Autodesk Fusion 360 part; units mm, degrees
note: some values were not read from the file. Set by a fixed rule: which sketch regions a step uses.
(part 17 of 20)
  spline S97 degree 5 poles (-21.1029, 22.7084) (-21.1018, 22.7059) (-21.0998, 22.7009) (-21.0967, 22.6934) (-21.0925, 22.6834) (-21.0873, 22.671) (-21.0822, 22.6586) (-21.077, 22.6462) (-21.0718, 22.6339) (-21.0666, 22.6217) (-21.0614, 22.6094) (-21.0562, 22.5972) (-21.051, 22.585) (-21.0458, 22.5729) (-21.0406, 22.5608) (-21.0354, 22.5487) (-21.0302, 22.5367) (-21.025, 22.5247) (-21.0198, 22.5127) (-21.0145, 22.5008) (-21.0093, 22.4889) (-21.0041, 22.4771) (-20.9989, 22.4653) (-20.9937, 22.4535) (-20.9884, 22.4417) (-20.9832, 22.43) (-20.978, 22.4184) (-20.9727, 22.4067) (-20.9675, 22.3951) (-20.9623, 22.3836) (-20.957, 22.3721) (-20.9518, 22.3606) (-20.9466, 22.3491) (-20.9413, 22.3377) (-20.9361, 22.3264) (-20.9308, 22.315) (-20.9256, 22.3037) (-20.9204, 22.2925) (-20.9151, 22.2812) (-20.9099, 22.2701) (-20.9046, 22.2589) (-20.8994, 22.2478) (-20.8942, 22.2367) (-20.8889, 22.2257) (-20.8837, 22.2147) (-20.8784, 22.2038) (-20.8732, 22.1928) (-20.868, 22.182) (-20.8627, 22.1711) (-20.8575, 22.1603) (-20.8523, 22.1496) (-20.847, 22.1388) (-20.8418, 22.1281) (-20.8366, 22.1175) (-20.8313, 22.1069) (-20.8261, 22.0963) (-20.8209, 22.0858) (-20.8157, 22.0753) (-20.8105, 22.0649) (-20.8052, 22.0544) (-20.8, 22.0441) (-20.7948, 22.0337) (-20.7896, 22.0235) (-20.7844, 22.0132) (-20.7792, 22.003) (-20.774, 21.9928) (-20.7688, 21.9827) (-20.7636, 21.9726) (-20.7584, 21.9625) (-20.7532, 21.9525) (-20.748, 21.9426) (-20.7429, 21.9326) (-20.7377, 21.9228) (-20.7325, 21.9129) (-20.7274, 21.9031) (-20.7222, 21.8933) (-20.717, 21.8836) (-20.7119, 21.8739) (-20.7067, 21.8643) (-20.7016, 21.8547) (-20.6965, 21.8451) (-20.6913, 21.8356) (-20.6862, 21.8261) (-20.6811, 21.8167) (-20.676, 21.8073) (-20.6709, 21.798) (-20.6658, 21.7887) (-20.6607, 21.7794) (-20.6556, 21.7702) (-20.6505, 21.761) (-20.6454, 21.7519) (-20.6404, 21.7428) (-20.6353, 21.7337) (-20.6303, 21.7247) (-20.6252, 21.7158) (-20.6202, 21.7068) (-20.6152, 21.698) (-20.6101, 21.6891) (-20.6051, 21.6803) (-20.6001, 21.6716) (-20.5951, 21.6629) (-20.5902, 21.6542) (-20.5852, 21.6456) (-20.5802, 21.6371) (-20.5753, 21.6285) (-20.5703, 21.6201) (-20.5654, 21.6116) (-20.5605, 21.6032) (-20.5555, 21.5949) (-20.5506, 21.5866) (-20.5457, 21.5783) (-20.5409, 21.5701) (-20.536, 21.5619) (-20.5311, 21.5538) (-20.5263, 21.5458) (-20.5214, 21.5377) (-20.5166, 21.5297) (-20.5118, 21.5218) (-20.507, 21.5139) (-20.5022, 21.5061) (-20.4974, 21.4983) (-20.4927, 21.4905) (-20.4879, 21.4828) (-20.4832, 21.4752) (-20.4784, 21.4676) (-20.4737, 21.46) (-20.469, 21.4525) (-20.4644, 21.445) (-20.4597, 21.4376) (-20.455, 21.4302) (-20.4504, 21.4229) (-20.4458, 21.4156) (-20.4412, 21.4084) (-20.4366, 21.4012) (-20.432, 21.3941) (-20.4274, 21.387) (-20.4229, 21.38) (-20.4184, 21.373) (-20.4139, 21.3661) (-20.4094, 21.3592) (-20.4049, 21.3523) (-20.4004, 21.3455) (-20.396, 21.3388) (-20.3916, 21.3321) (-20.3872, 21.3255) (-20.3828, 21.3189) (-20.3784, 21.3124) (-20.3741, 21.3059) (-20.3698, 21.2995) (-20.3655, 21.2931) (-20.3612, 21.2867) (-20.3569, 21.2805) (-20.3527, 21.2742) (-20.3484, 21.2681) (-20.3442, 21.2619) (-20.3401, 21.2559) (-20.3359, 21.2498) (-20.3318, 21.2439) (-20.3277, 21.238) (-20.3236, 21.2321) (-20.3195, 21.2263) (-20.3155, 21.2205) (-20.3115, 21.2148) (-20.3075, 21.2092) (-20.3035, 21.2036) (-20.2996, 21.1981) (-20.2956, 21.1926) (-20.2918, 21.1871) (-20.2879, 21.1818) (-20.2841, 21.1764) (-20.2802, 21.1712) (-20.2765, 21.166) (-20.2727, 21.1608) (-20.269, 21.1557) (-20.2653, 21.1507) (-20.2616, 21.1457) (-20.258, 21.1408) (-20.2544, 21.1359) (-20.2508, 21.1311) (-20.2472, 21.1263) (-20.2437, 21.1216) (-20.2402, 21.117) (-20.2368, 21.1124) (-20.2333, 21.1079) (-20.23, 21.1034) (-20.2266, 21.099) (-20.2233, 21.0947) (-20.22, 21.0904) (-20.2167, 21.0862) (-20.2135, 21.082) (-20.2103, 21.0779) (-20.2072, 21.0739) (-20.2041, 21.0699) (-20.201, 21.066) (-20.198, 21.0621) (-20.195, 21.0583) (-20.192, 21.0546) (-20.1891, 21.0509) (-20.1862, 21.0473) (-20.1834, 21.0437) (-20.1806, 21.0403) (-20.1778, 21.0368) (-20.1751, 21.0335) (-20.1724, 21.0302) (-20.1698, 21.027) (-20.1672, 21.0238) (-20.1647, 21.0207) (-20.1622, 21.0177) (-20.1597, 21.0148) (-20.1573, 21.0119) (-20.155, 21.009) (-20.1527, 21.0063) (-20.1504, 21.0036) (-20.1482, 21.001) (-20.1461, 20.9984) (-20.144, 20.996) (-20.1419, 20.9936) (-20.1399, 20.9912) (-20.138, 20.989) (-20.1361, 20.9868) (-20.1343, 20.9847) (-20.1325, 20.9826) (-20.1308, 20.9806) (-20.1291, 20.9787) (-20.1275, 20.9769) (-20.126, 20.9752) (-20.1245, 20.9735) (-20.123, 20.9719) (-20.1217, 20.9704) (-20.1204, 20.9689) (-20.1192, 20.9675) (-20.118, 20.9663) (-20.1169, 20.9651) (-20.1159, 20.9639) (-20.1149, 20.9629) (-20.114, 20.9619) (-20.1132, 20.961) (-20.1125, 20.9602) (-20.1118, 20.9595) (-20.1112, 20.9589) (-20.1107, 20.9583) (-20.1104, 20.958) (-20.1102, 20.9577) (-20.11, 20.9576) (-20.11, 20.9575) knots -1 -1 -1 -1 -1 -1 -0.99583333 -0.99166667 -0.9875 -0.98333333 -0.97916667 -0.975 -0.97083333 -0.96666667 -0.9625 -0.95833333 -0.95416667 -0.95 -0.94583333 -0.94166667 -0.9375 -0.93333333 -0.92916667 -0.925 -0.92083333 -0.91666667 -0.9125 -0.90833333 -0.90416667 -0.9 -0.89583333 -0.89166667 -0.8875 -0.88333333 -0.87916667 -0.875 -0.87083333 -0.86666667 -0.8625 -0.85833333 -0.85416667 -0.85 -0.84583333 -0.84166667 -0.8375 -0.83333333 -0.82916667 -0.825 -0.82083333 -0.81666667 -0.8125 -0.80833333 -0.80416667 -0.8 -0.79583333 -0.79166667 -0.7875 -0.78333333 -0.77916667 -0.775 -0.77083333 -0.76666667 -0.7625 -0.75833333 -0.75416667 -0.75 -0.74583333 -0.74166667 -0.7375 -0.73333333 -0.72916667 -0.725 -0.72083333 -0.71666667 -0.7125 -0.70833333 -0.70416667 -0.7 -0.69583333 -0.69166667 -0.6875 -0.68333333 -0.67916667 -0.675 -0.67083333 -0.66666667 -0.6625 -0.65833333 -0.65416667 -0.65 -0.64583333 -0.64166667 -0.6375 -0.63333333 -0.62916667 -0.625 -0.62083333 -0.61666667 -0.6125 -0.60833333 -0.60416667 -0.6 -0.59583333 -0.59166667 -0.5875 -0.58333333 -0.57916667 -0.575 -0.57083333 -0.56666667 -0.5625 -0.55833333 -0.55416667 -0.55 -0.54583333 -0.54166667 -0.5375 -0.53333333 -0.52916667 -0.525 -0.52083333 -0.51666667 -0.5125 -0.50833333 -0.50416667 -0.5 -0.49583333 -0.49166667 -0.4875 -0.48333333 -0.47916667 -0.475 -0.47083333 -0.46666667 -0.4625 -0.45833333 -0.45416667 -0.45 -0.44583333 -0.44166667 -0.4375 -0.43333333 -0.42916667 -0.425 -0.42083333 -0.41666667 -0.4125 -0.40833333 -0.40416667 -0.4 -0.39583333 -0.39166667 -0.3875 -0.38333333 -0.37916667 -0.375 -0.37083333 -0.36666667 -0.3625 -0.35833333 -0.35416667 -0.35 -0.34583333 -0.34166667 -0.3375 -0.33333333 -0.32916667 -0.325 -0.32083333 -0.31666667 -0.3125 -0.30833333 -0.30416667 -0.3 -0.29583333 -0.29166667 -0.2875 -0.28333333 -0.27916667 -0.275 -0.27083333 -0.26666667 -0.2625 -0.25833333 -0.25416667 -0.25 -0.24583333 -0.24166667 -0.2375 -0.23333333 -0.22916667 -0.225 -0.22083333 -0.21666667 -0.2125 -0.20833333 -0.20416667 -0.2 -0.19583333 -0.19166667 -0.1875 -0.18333333 -0.17916667 -0.175 -0.17083333 -0.16666667 -0.1625 -0.15833333 -0.15416667 -0.15 -0.14583333 -0.14166667 -0.1375 -0.13333333 -0.12916667 -0.125 -0.12083333 -0.11666667 -0.1125 -0.10833333 -0.10416667 -0.1 -0.09583333 -0.09166667 -0.0875 -0.08333333 -0.07916667 -0.075 -0.07083333 -0.06666667 -0.0625 -0.05833333 -0.05416667 -0.05 -0.04583333 -0.04166667 -0.0375 -0.03333333 -0.02916667 -0.025 -0.02083333 -0.01666667 -0.0125 -0.00833333 -0.00416667 0 0 0 0 0 0
  spline S98 degree 5 poles (30.9962, 0.4876) (30.9936, 0.4885) (30.9885, 0.4903) (30.9809, 0.493) (30.9707, 0.4966) (30.958, 0.5011) (30.9453, 0.5055) (30.9327, 0.5099) (30.9201, 0.5143) (30.9075, 0.5187) (30.8949, 0.523) (30.8823, 0.5273) (30.8698, 0.5316) (30.8573, 0.5359) (30.8448, 0.5401) (30.8324, 0.5443) (30.82, 0.5485) (30.8076, 0.5526) (30.7952, 0.5568) (30.7828, 0.5609) (30.7705, 0.5649) (30.7582, 0.569) (30.7459, 0.573) (30.7337, 0.577) (30.7215, 0.581) (30.7093, 0.5849) (30.6971, 0.5889) (30.685, 0.5927) (30.6728, 0.5966) (30.6607, 0.6005) (30.6487, 0.6043) (30.6366, 0.6081) (30.6246, 0.6118) (30.6126, 0.6156) (30.6007, 0.6193) (30.5888, 0.623) (30.5769, 0.6267) (30.565, 0.6303) (30.5531, 0.6339) (30.5413, 0.6375) (30.5295, 0.6411) (30.5178, 0.6446) (30.506, 0.6481) (30.4943, 0.6516) (30.4827, 0.6551) (30.471, 0.6585) (30.4594, 0.6619) (30.4478, 0.6653) (30.4362, 0.6687) (30.4247, 0.672) (30.4132, 0.6753) (30.4017, 0.6786) (30.3903, 0.6819) (30.3789, 0.6851) (30.3675, 0.6883) (30.3562, 0.6915) (30.3448, 0.6947) (30.3336, 0.6978) (30.3223, 0.7009) (30.3111, 0.704) (30.2999, 0.7071) (30.2887, 0.7101) (30.2776, 0.7131) (30.2665, 0.7161) (30.2554, 0.7191) (30.2444, 0.722) (30.2334, 0.7249) (30.2224, 0.7278) (30.2114, 0.7307) (30.2005, 0.7335) (30.1897, 0.7364) (30.1788, 0.7391) (30.168, 0.7419) (30.1572, 0.7447) (30.1465, 0.7474) (30.1358, 0.7501) (30.1251, 0.7528) (30.1145, 0.7554) (30.1038, 0.758) (30.0933, 0.7606) (30.0827, 0.7632) (30.0722, 0.7658) (30.0618, 0.7683) (30.0513, 0.7708) (30.0409, 0.7733) (30.0306, 0.7758) (30.0202, 0.7782) (30.0099, 0.7806) (29.9997, 0.783) (29.9895, 0.7854) (29.9793, 0.7877) (29.9691, 0.79) (29.959, 0.7923) (29.949, 0.7946) (29.9389, 0.7969) (29.9289, 0.7991) (29.919, 0.8013) (29.909, 0.8035) (29.8992, 0.8056) (29.8893, 0.8078) (29.8795, 0.8099) (29.8697, 0.812) (29.86, 0.814) (29.8503, 0.8161) (29.8407, 0.8181) (29.8311, 0.8201) (29.8215, 0.8221) (29.812, 0.824) (29.8025, 0.8259) (29.793, 0.8279) (29.7836, 0.8297) (29.7742, 0.8316) (29.7649, 0.8334) (29.7556, 0.8353) (29.7464, 0.8371) (29.7372, 0.8388) (29.728, 0.8406) (29.7189, 0.8423) (29.7098, 0.844) (29.7008, 0.8457) (29.6918, 0.8474) (29.6828, 0.849) (29.6739, 0.8507) (29.6651, 0.8523) (29.6563, 0.8538) (29.6475, 0.8554) (29.6388, 0.8569) (29.6301, 0.8585) (29.6214, 0.86) (29.6128, 0.8614) (29.6043, 0.8629) (29.5958, 0.8643) (29.5873, 0.8657) (29.5789, 0.8671) (29.5706, 0.8685) (29.5623, 0.8698) (29.554, 0.8712) (29.5458, 0.8725) (29.5376, 0.8738) (29.5295, 0.875) (29.5214, 0.8763) (29.5134, 0.8775) (29.5054, 0.8787) (29.4975, 0.8799) (29.4896, 0.8811) (29.4818, 0.8822) (29.474, 0.8834) (29.4663, 0.8845) (29.4586, 0.8856) (29.451, 0.8866) (29.4434, 0.8877) (29.4359, 0.8887) (29.4284, 0.8897) (29.421, 0.8907) (29.4137, 0.8917) (29.4063, 0.8927) (29.3991, 0.8936) (29.3919, 0.8945) (29.3847, 0.8954) (29.3777, 0.8963) (29.3706, 0.8972) (29.3636, 0.898) (29.3567, 0.8989) (29.3498, 0.8997) (29.343, 0.9005) (29.3363, 0.9012) (29.3296, 0.902) (29.323, 0.9027) (29.3164, 0.9035) (29.3099, 0.9042) (29.3034, 0.9049) (29.297, 0.9055) (29.2906, 0.9062) (29.2844, 0.9068) (29.2781, 0.9075) (29.272, 0.9081) (29.2659, 0.9087) (29.2599, 0.9092) (29.2539, 0.9098) (29.248, 0.9103) (29.2421, 0.9109) (29.2363, 0.9114) (29.2306, 0.9119) (29.225, 0.9124) (29.2194, 0.9128) (29.2139, 0.9133) (29.2084, 0.9137) (29.203, 0.9141) (29.1977, 0.9146) (29.1925, 0.915) (29.1873, 0.9153) (29.1822, 0.9157) (29.1771, 0.9161) (29.1722, 0.9164) (29.1673, 0.9167) (29.1624, 0.917) (29.1577, 0.9173) (29.153, 0.9176) (29.1484, 0.9179) (29.1439, 0.9182) (29.1394, 0.9184) (29.135, 0.9186) (29.1307, 0.9189) (29.1265, 0.9191) (29.1223, 0.9193) (29.1183, 0.9195) (29.1143, 0.9197) (29.1103, 0.9198) (29.1065, 0.92) (29.1028, 0.9201) (29.0991, 0.9203) (29.0955, 0.9204) (29.092, 0.9205) (29.0886, 0.9206) (29.0852, 0.9208) (29.082, 0.9208) (29.0788, 0.9209) (29.0758, 0.921) (29.0728, 0.9211) (29.0699, 0.9211) (29.0671, 0.9212) (29.0644, 0.9212) (29.0618, 0.9213) (29.0592, 0.9213) (29.0568, 0.9214) (29.0545, 0.9214) (29.0522, 0.9214) (29.0501, 0.9214) (29.0481, 0.9214) (29.0461, 0.9214) (29.0443, 0.9214) (29.0425, 0.9214) (29.0409, 0.9214) (29.0394, 0.9214) (29.038, 0.9214) (29.0367, 0.9214) (29.0355, 0.9214) (29.0344, 0.9214) (29.0334, 0.9213) (29.0325, 0.9213) (29.0318, 0.9213) (29.0313, 0.9213) (29.0309, 0.9213) (29.0307, 0.9213) (29.0307, 0.9213) knots -1 -1 -1 -1 -1 -1 -0.99583333 -0.99166667 -0.9875 -0.98333333 -0.97916667 -0.975 -0.97083333 -0.96666667 -0.9625 -0.95833333 -0.95416667 -0.95 -0.94583333 -0.94166667 -0.9375 -0.93333333 -0.92916667 -0.925 -0.92083333 -0.91666667 -0.9125 -0.90833333 -0.90416667 -0.9 -0.89583333 -0.89166667 -0.8875 -0.88333333 -0.87916667 -0.875 -0.87083333 -0.86666667 -0.8625 -0.85833333 -0.85416667 -0.85 -0.84583333 -0.84166667 -0.8375 -0.83333333 -0.82916667 -0.825 -0.82083333 -0.81666667 -0.8125 -0.80833333 -0.80416667 -0.8 -0.79583333 -0.79166667 -0.7875 -0.78333333 -0.77916667 -0.775 -0.77083333 -0.76666667 -0.7625 -0.75833333 -0.75416667 -0.75 -0.74583333 -0.74166667 -0.7375 -0.73333333 -0.72916667 -0.725 -0.72083333 -0.71666667 -0.7125 -0.70833333 -0.70416667 -0.7 -0.69583333 -0.69166667 -0.6875 -0.68333333 -0.67916667 -0.675 -0.67083333 -0.66666667 -0.6625 -0.65833333 -0.65416667 -0.65 -0.64583333 -0.64166667 -0.6375 -0.63333333 -0.62916667 -0.625 -0.62083333 -0.61666667 -0.6125 -0.60833333 -0.60416667 -0.6 -0.59583333 -0.59166667 -0.5875 -0.58333333 -0.57916667 -0.575 -0.57083333 -0.56666667 -0.5625 -0.55833333 -0.55416667 -0.55 -0.54583333 -0.54166667 -0.5375 -0.53333333 -0.52916667 -0.525 -0.52083333 -0.51666667 -0.5125 -0.50833333 -0.50416667 -0.5 -0.49583333 -0.49166667 -0.4875 -0.48333333 -0.47916667 -0.475 -0.47083333 -0.46666667 -0.4625 -0.45833333 -0.45416667 -0.45 -0.44583333 -0.44166667 -0.4375 -0.43333333 -0.42916667 -0.425 -0.42083333 -0.41666667 -0.4125 -0.40833333 -0.40416667 -0.4 -0.39583333 -0.39166667 -0.3875 -0.38333333 -0.37916667 -0.375 -0.37083333 -0.36666667 -0.3625 -0.35833333 -0.35416667 -0.35 -0.34583333 -0.34166667 -0.3375 -0.33333333 -0.32916667 -0.325 -0.32083333 -0.31666667 -0.3125 -0.30833333 -0.30416667 -0.3 -0.29583333 -0.29166667 -0.2875 -0.28333333 -0.27916667 -0.275 -0.27083333 -0.26666667 -0.2625 -0.25833333 -0.25416667 -0.25 -0.24583333 -0.24166667 -0.2375 -0.23333333 -0.22916667 -0.225 -0.22083333 -0.21666667 -0.2125 -0.20833333 -0.20416667 -0.2 -0.19583333 -0.19166667 -0.1875 -0.18333333 -0.17916667 -0.175 -0.17083333 -0.16666667 -0.1625 -0.15833333 -0.15416667 -0.15 -0.14583333 -0.14166667 -0.1375 -0.13333333 -0.12916667 -0.125 -0.12083333 -0.11666667 -0.1125 -0.10833333 -0.10416667 -0.1 -0.09583333 -0.09166667 -0.0875 -0.08333333 -0.07916667 -0.075 -0.07083333 -0.06666667 -0.0625 -0.05833333 -0.05416667 -0.05 -0.04583333 -0.04166667 -0.0375 -0.03333333 -0.02916667 -0.025 -0.02083333 -0.01666667 -0.0125 -0.00833333 -0.00416667 0 0 0 0 0 0
  arc A99 (-22.7084, 21.1029) -> (-23.3609, 20.3781) centre (0, 0) ccw
  spline S99 degree 5 poles (-12.6495, -26.1461) (-12.6495, -26.1462) (-12.6496, -26.1464) (-12.6497, -26.1467) (-12.65, -26.1471) (-12.6503, -26.1478) (-12.6506, -26.1486) (-12.651, -26.1495) (-12.6515, -26.1504) (-12.652, -26.1515) (-12.6526, -26.1527) (-12.6531, -26.154) (-12.6538, -26.1554) (-12.6544, -26.1569) (-12.6551, -26.1585) (-12.6559, -26.1602) (-12.6567, -26.1619) (-12.6575, -26.1638) (-12.6583, -26.1658) (-12.6592, -26.1678) (-12.6602, -26.17) (-12.6611, -26.1722) (-12.6621, -26.1745) (-12.6631, -26.1769) (-12.6642, -26.1794) (-12.6653, -26.182) (-12.6664, -26.1847) (-12.6676, -26.1874) (-12.6687, -26.1903) (-12.6699, -26.1932) (-12.6712, -26.1962) (-12.6724, -26.1993) (-12.6737, -26.2024) (-12.675, -26.2057) (-12.6764, -26.209) (-12.6778, -26.2124) (-12.6791, -26.2159) (-12.6806, -26.2195) (-12.682, -26.2231) (-12.6834, -26.2269) (-12.6849, -26.2307) (-12.6864, -26.2345) (-12.688, -26.2385) (-12.6895, -26.2425) (-12.6911, -26.2466) (-12.6927, -26.2508) (-12.6943, -26.255) (-12.6959, -26.2594) (-12.6975, -26.2638) (-12.6992, -26.2682) (-12.7009, -26.2728) (-12.7026, -26.2774) (-12.7043, -26.282) (-12.706, -26.2868) (-12.7077, -26.2916) (-12.7095, -26.2965) (-12.7113, -26.3015) (-12.7131, -26.3065) (-12.7149, -26.3116) (-12.7167, -26.3167) (-12.7185, -26.322) (-12.7204, -26.3273) (-12.7222, -26.3326) (-12.7241, -26.338) (-12.726, -26.3435) (-12.7279, -26.3491) (-12.7298, -26.3547) (-12.7317, -26.3604) (-12.7336, -26.3661) (-12.7356, -26.3719) (-12.7375, -26.3778) (-12.7395, -26.3837) (-12.7414, -26.3897) (-12.7434, -26.3958) (-12.7454, -26.4019) (-12.7474, -26.4081) (-12.7494, -26.4144) (-12.7514, -26.4207) (-12.7534, -26.427) (-12.7555, -26.4335) (-12.7575, -26.4399) (-12.7596, -26.4465) (-12.7616, -26.4531) (-12.7637, -26.4598) (-12.7657, -26.4665) (-12.7678, -26.4733) (-12.7699, -26.4801) (-12.772, -26.487) (-12.774, -26.4939) (-12.7761, -26.5009) (-12.7782, -26.508) (-12.7803, -26.5151) (-12.7824, -26.5223) (-12.7845, -26.5296) (-12.7867, -26.5368) (-12.7888, -26.5442) (-12.7909, -26.5516) (-12.793, -26.559) (-12.7952, -26.5665) (-12.7973, -26.5741) (-12.7994, -26.5817) (-12.8016, -26.5894) (-12.8037, -26.5971) (-12.8058, -26.6049) (-12.808, -26.6127) (-12.8101, -26.6206) (-12.8123, -26.6286) (-12.8144, -26.6365) (-12.8166, -26.6446) (-12.8187, -26.6527) (-12.8208, -26.6608) (-12.823, -26.669) (-12.8251, -26.6773) (-12.8273, -26.6856) (-12.8294, -26.6939) (-12.8316, -26.7023) (-12.8337, -26.7108) (-12.8359, -26.7193) (-12.838, -26.7278) (-12.8402, -26.7364) (-12.8423, -26.7451) (-12.8445, -26.7537) (-12.8466, -26.7625) (-12.8487, -26.7713) (-12.8509, -26.7801) (-12.853, -26.789) (-12.8551, -26.798) (-12.8573, -26.8069) (-12.8594, -26.816) (-12.8615, -26.8251) (-12.8636, -26.8342) (-12.8658, -26.8434) (-12.8679, -26.8526) (-12.87, -26.8619) (-12.8721, -26.8712) (-12.8742, -26.8806) (-12.8763, -26.89) (-12.8784, -26.8994) (-12.8805, -26.9089) (-12.8826, -26.9185) (-12.8847, -26.9281) (-12.8867, -26.9377) (-12.8888, -26.9474) (-12.8909, -26.9571) (-12.8929, -26.9669) (-12.895, -26.9767) (-12.8971, -26.9866) (-12.8991, -26.9965) (-12.9011, -27.0064) (-12.9032, -27.0164) (-12.9052, -27.0265) (-12.9072, -27.0365) (-12.9093, -27.0467) (-12.9113, -27.0568) (-12.9133, -27.0671) (-12.9153, -27.0773) (-12.9173, -27.0876) (-12.9193, -27.0979) (-12.9213, -27.1083) (-12.9232, -27.1188) (-12.9252, -27.1292) (-12.9272, -27.1397) (-12.9291, -27.1503) (-12.9311, -27.1609) (-12.933, -27.1715) (-12.9349, -27.1822) (-12.9368, -27.1929) (-12.9388, -27.2037) (-12.9407, -27.2145) (-12.9426, -27.2253) (-12.9445, -27.2362) (-12.9463, -27.2471) (-12.9482, -27.2581) (-12.9501, -27.2691) (-12.9519, -27.2801) (-12.9538, -27.2912) (-12.9556, -27.3023) (-12.9574, -27.3135) (-12.9593, -27.3247) (-12.9611, -27.3359) (-12.9629, -27.3472) (-12.9647, -27.3585) (-12.9665, -27.3699) (-12.9682, -27.3813) (-12.97, -27.3927) (-12.9718, -27.4042) (-12.9735, -27.4157) (-12.9752, -27.4273) (-12.977, -27.4388) (-12.9787, -27.4505) (-12.9804, -27.4621) (-12.9821, -27.4738) (-12.9838, -27.4856) (-12.9854, -27.4974) (-12.9871, -27.5092) (-12.9887, -27.521) (-12.9904, -27.5329) (-12.992, -27.5449) (-12.9936, -27.5568) (-12.9952, -27.5688) (-12.9968, -27.5809) (-12.9984, -27.5929) (-13, -27.605) (-13.0016, -27.6172) (-13.0031, -27.6294) (-13.0047, -27.6416) (-13.0062, -27.6539) (-13.0077, -27.6661) (-13.0092, -27.6785) (-13.0107, -27.6908) (-13.0122, -27.7032) (-13.0136, -27.7157) (-13.0151, -27.7281) (-13.0165, -27.7406) (-13.018, -27.7532) (-13.0194, -27.7658) (-13.0208, -27.7784) (-13.0222, -27.791) (-13.0236, -27.8037) (-13.0249, -27.8164) (-13.0263, -27.8291) (-13.0276, -27.8419) (-13.029, -27.8547) (-13.0303, -27.8676) (-13.0316, -27.8805) (-13.0329, -27.8934) (-13.0342, -27.9063) (-13.0354, -27.9193) (-13.0367, -27.9323) (-13.0379, -27.9454) (-13.0391, -27.9585) (-13.0404, -27.9716) (-13.0415, -27.9848) (-13.0427, -27.9979) (-13.0439, -28.0112) (-13.0451, -28.0244) (-13.0462, -28.0377) (-13.0473, -28.051) (-13.0484, -28.0644) (-13.0495, -28.0777) (-13.0506, -28.0911) (-13.0515, -28.1019) (-13.0521, -28.11) (-13.0525, -28.1154) (-13.0527, -28.1181) knots 0 0 0 0 0 0 0.00416667 0.00833333 0.0125 0.01666667 0.02083333 0.025 0.02916667 0.03333333 0.0375 0.04166667 0.04583333 0.05 0.05416667 0.05833333 0.0625 0.06666667 0.07083333 0.075 0.07916667 0.08333333 0.0875 0.09166667 0.09583333 0.1 0.10416667 0.10833333 0.1125 0.11666667 0.12083333 0.125 0.12916667 0.13333333 0.1375 0.14166667 0.14583333 0.15 0.15416667 0.15833333 0.1625 0.16666667 0.17083333 0.175 0.17916667 0.18333333 0.1875 0.19166667 0.19583333 0.2 0.20416667 0.20833333 0.2125 0.21666667 0.22083333 0.225 0.22916667 0.23333333 0.2375 0.24166667 0.24583333 0.25 0.25416667 0.25833333 0.2625 0.26666667 0.27083333 0.275 0.27916667 0.28333333 0.2875 0.29166667 0.29583333 0.3 0.30416667 0.30833333 0.3125 0.31666667 0.32083333 0.325 0.32916667 0.33333333 0.3375 0.34166667 0.34583333 0.35 0.35416667 0.35833333 0.3625 0.36666667 0.37083333 0.375 0.37916667 0.38333333 0.3875 0.39166667 0.39583333 0.4 0.40416667 0.40833333 0.4125 0.41666667 0.42083333 0.425 0.42916667 0.43333333 0.4375 0.44166667 0.44583333 0.45 0.45416667 0.45833333 0.4625 0.46666667 0.47083333 0.475 0.47916667 0.48333333 0.4875 0.49166667 0.49583333 0.5 0.50416667 0.50833333 0.5125 0.51666667 0.52083333 0.525 0.52916667 0.53333333 0.5375 0.54166667 0.54583333 0.55 0.55416667 0.55833333 0.5625 0.56666667 0.57083333 0.575 0.57916667 0.58333333 0.5875 0.59166667 0.59583333 0.6 0.60416667 0.60833333 0.6125 0.61666667 0.62083333 0.625 0.62916667 0.63333333 0.6375 0.64166667 0.64583333 0.65 0.65416667 0.65833333 0.6625 0.66666667 0.67083333 0.675 0.67916667 0.68333333 0.6875 0.69166667 0.69583333 0.7 0.70416667 0.70833333 0.7125 0.71666667 0.72083333 0.725 0.72916667 0.73333333 0.7375 0.74166667 0.74583333 0.75 0.75416667 0.75833333 0.7625 0.76666667 0.77083333 0.775 0.77916667 0.78333333 0.7875 0.79166667 0.79583333 0.8 0.80416667 0.80833333 0.8125 0.81666667 0.82083333 0.825 0.82916667 0.83333333 0.8375 0.84166667 0.84583333 0.85 0.85416667 0.85833333 0.8625 0.86666667 0.87083333 0.875 0.87916667 0.88333333 0.8875 0.89166667 0.89583333 0.9 0.90416667 0.90833333 0.9125 0.91666667 0.92083333 0.925 0.92916667 0.93333333 0.9375 0.94166667 0.94583333 0.95 0.95416667 0.95833333 0.9625 0.96666667 0.97083333 0.975 0.97916667 0.98333333 0.9875 0.99166667 0.99583333 1 1 1 1 1 1
  arc A100 (30.8773, 2.755) -> (30.7754, 3.7249) centre (0, 0) ccw
  line L194 (-18.7401, -22.1898) -> (-18.5501, -21.9649)
  line L195 (28.7753, 3.9508) -> (28.7745, 3.9507)
  circle A101 centre (0, 0) radius 4
  line L196 (28.9671, 2.1182) -> (28.9679, 2.1183)
  circle A102 centre (10, 0) radius 1.7
  arc A103 (-13.578, -25.3417) -> (-12.5209, -25.8803) centre (0, 0) ccw
  spline S100 degree 5 poles (-23.3609, 20.3781) (-23.3596, 20.3757) (-23.3571, 20.371) (-23.3532, 20.3639) (-23.348, 20.3544) (-23.3416, 20.3426) (-23.3351, 20.3308) (-23.3287, 20.319) (-23.3222, 20.3073) (-23.3158, 20.2957) (-23.3094, 20.284) (-23.3029, 20.2724) (-23.2965, 20.2609) (-23.29, 20.2493) (-23.2836, 20.2379) (-23.2771, 20.2264) (-23.2707, 20.215) (-23.2643, 20.2036) (-23.2578, 20.1922) (-23.2514, 20.1809) (-23.245, 20.1697) (-23.2385, 20.1584) (-23.2321, 20.1472) (-23.2257, 20.136) (-23.2193, 20.1249) (-23.2128, 20.1138) (-23.2064, 20.1028) (-23.2, 20.0917) (-23.1936, 20.0808) (-23.1872, 20.0698) (-23.1807, 20.0589) (-23.1743, 20.048) (-23.1679, 20.0372) (-23.1615, 20.0264) (-23.1551, 20.0156) (-23.1487, 20.0049) (-23.1423, 19.9942) (-23.136, 19.9836) (-23.1296, 19.973) (-23.1232, 19.9624) (-23.1168, 19.9518) (-23.1104, 19.9413) (-23.1041, 19.9309) (-23.0977, 19.9205) (-23.0914, 19.9101) (-23.085, 19.8997) (-23.0786, 19.8894) (-23.0723, 19.8791) (-23.066, 19.8689) (-23.0596, 19.8587) (-23.0533, 19.8486) (-23.047, 19.8384) (-23.0406, 19.8284) (-23.0343, 19.8183) (-23.028, 19.8083) (-23.0217, 19.7984) (-23.0154, 19.7884) (-23.0091, 19.7785) (-23.0029, 19.7687) (-22.9966, 19.7589) (-22.9903, 19.7491) (-22.984, 19.7394) (-22.9778, 19.7297) (-22.9715, 19.72) (-22.9653, 19.7104) (-22.9591, 19.7009) (-22.9528, 19.6913) (-22.9466, 19.6818) (-22.9404, 19.6724) (-22.9342, 19.663) (-22.928, 19.6536) (-22.9218, 19.6443) (-22.9156, 19.635) (-22.9095, 19.6257) (-22.9033, 19.6165) (-22.8971, 19.6073) (-22.891, 19.5982) (-22.8849, 19.5891) (-22.8787, 19.5801) (-22.8726, 19.5711) (-22.8665, 19.5621) (-22.8604, 19.5532) (-22.8543, 19.5443) (-22.8483, 19.5354) (-22.8422, 19.5266) (-22.8361, 19.5179) (-22.8301, 19.5091) (-22.8241, 19.5005) (-22.818, 19.4918) (-22.812, 19.4832) (-22.806, 19.4747) (-22.8, 19.4662) (-22.7941, 19.4577) (-22.7881, 19.4493) (-22.7822, 19.4409) (-22.7762, 19.4325) (-22.7703, 19.4242) (-22.7644, 19.416) (-22.7585, 19.4078) (-22.7526, 19.3996) (-22.7467, 19.3914) (-22.7408, 19.3834) (-22.735, 19.3753) (-22.7292, 19.3673) (-22.7233, 19.3593) (-22.7175, 19.3514) (-22.7118, 19.3436) (-22.706, 19.3357) (-22.7002, 19.3279) (-22.6945, 19.3202) (-22.6887, 19.3125) (-22.683, 19.3048) (-22.6773, 19.2972) (-22.6716, 19.2897) (-22.666, 19.2821) (-22.6603, 19.2747) (-22.6547, 19.2672) (-22.6491, 19.2598) (-22.6435, 19.2525) (-22.6379, 19.2452) (-22.6323, 19.2379) (-22.6268, 19.2307) (-22.6212, 19.2236) (-22.6157, 19.2165) (-22.6102, 19.2094) (-22.6048, 19.2024) (-22.5993, 19.1954) (-22.5939, 19.1884) (-22.5884, 19.1815) (-22.583, 19.1747) (-22.5777, 19.1679) (-22.5723, 19.1611) (-22.567, 19.1544) (-22.5617, 19.1478) (-22.5564, 19.1412) (-22.5511, 19.1346) (-22.5458, 19.1281) (-22.5406, 19.1216) (-22.5354, 19.1152) (-22.5302, 19.1088) (-22.525, 19.1025) (-22.5199, 19.0962) (-22.5148, 19.09) (-22.5097, 19.0838) (-22.5046, 19.0776) (-22.4996, 19.0715) (-22.4945, 19.0655) (-22.4895, 19.0595) (-22.4846, 19.0536) (-22.4796, 19.0477) (-22.4747, 19.0418) (-22.4698, 19.036) (-22.4649, 19.0303) (-22.4601, 19.0246) (-22.4553, 19.0189) (-22.4505, 19.0133) (-22.4457, 19.0077) (-22.441, 19.0022) (-22.4363, 18.9968) (-22.4316, 18.9914) (-22.427, 18.986) (-22.4223, 18.9807) (-22.4177, 18.9755) (-22.4132, 18.9703) (-22.4087, 18.9651) (-22.4042, 18.96) (-22.3997, 18.955) (-22.3953, 18.95) (-22.3909, 18.9451) (-22.3865, 18.9402) (-22.3821, 18.9353) (-22.3778, 18.9306) (-22.3736, 18.9258) (-22.3693, 18.9211) (-22.3651, 18.9165) (-22.3609, 18.9119) (-22.3568, 18.9074) (-22.3527, 18.903) (-22.3486, 18.8986) (-22.3446, 18.8942) (-22.3406, 18.8899) (-22.3367, 18.8856) (-22.3328, 18.8814) (-22.3289, 18.8773) (-22.325, 18.8732) (-22.3212, 18.8692) (-22.3175, 18.8652) (-22.3138, 18.8613) (-22.3101, 18.8574) (-22.3065, 18.8536) (-22.3029, 18.8499) (-22.2993, 18.8462) (-22.2958, 18.8426) (-22.2923, 18.839) (-22.2889, 18.8355) (-22.2855, 18.832) (-22.2822, 18.8286) (-22.2789, 18.8252) (-22.2757, 18.822) (-22.2725, 18.8187) (-22.2693, 18.8156) (-22.2662, 18.8124) (-22.2632, 18.8094) (-22.2602, 18.8064) (-22.2572, 18.8035) (-22.2543, 18.8006) (-22.2515, 18.7978) (-22.2487, 18.7951) (-22.2459, 18.7924) (-22.2433, 18.7897) (-22.2406, 18.7872) (-22.238, 18.7847) (-22.2355, 18.7823) (-22.2331, 18.7799) (-22.2307, 18.7776) (-22.2283, 18.7753) (-22.226, 18.7732) (-22.2238, 18.771) (-22.2216, 18.769) (-22.2195, 18.767) (-22.2175, 18.7651) (-22.2155, 18.7632) (-22.2136, 18.7615) (-22.2117, 18.7597) (-22.2099, 18.7581) (-22.2082, 18.7565) (-22.2066, 18.755) (-22.205, 18.7536) (-22.2035, 18.7522) (-22.202, 18.7509) (-22.2007, 18.7497) (-22.1994, 18.7485) (-22.1982, 18.7474) (-22.197, 18.7464) (-22.196, 18.7455) (-22.195, 18.7446) (-22.1941, 18.7438) (-22.1933, 18.7431) (-22.1925, 18.7424) (-22.1919, 18.7419) (-22.1913, 18.7414) (-22.1909, 18.741) (-22.1907, 18.7408) (-22.1905, 18.7407) (-22.1904, 18.7406) knots -1 -1 -1 -1 -1 -1 -0.99583333 -0.99166667 -0.9875 -0.98333333 -0.97916667 -0.975 -0.97083333 -0.96666667 -0.9625 -0.95833333 -0.95416667 -0.95 -0.94583333 -0.94166667 -0.9375 -0.93333333 -0.92916667 -0.925 -0.92083333 -0.91666667 -0.9125 -0.90833333 -0.90416667 -0.9 -0.89583333 -0.89166667 -0.8875 -0.88333333 -0.87916667 -0.875 -0.87083333 -0.86666667 -0.8625 -0.85833333 -0.85416667 -0.85 -0.84583333 -0.84166667 -0.8375 -0.83333333 -0.82916667 -0.825 -0.82083333 -0.81666667 -0.8125 -0.80833333 -0.80416667 -0.8 -0.79583333 -0.79166667 -0.7875 -0.78333333 -0.77916667 -0.775 -0.77083333 -0.76666667 -0.7625 -0.75833333 -0.75416667 -0.75 -0.74583333 -0.74166667 -0.7375 -0.73333333 -0.72916667 -0.725 -0.72083333 -0.71666667 -0.7125 -0.70833333 -0.70416667 -0.7 -0.69583333 -0.69166667 -0.6875 -0.68333333 -0.67916667 -0.675 -0.67083333 -0.66666667 -0.6625 -0.65833333 -0.65416667 -0.65 -0.64583333 -0.64166667 -0.6375 -0.63333333 -0.62916667 -0.625 -0.62083333 -0.61666667 -0.6125 -0.60833333 -0.60416667 -0.6 -0.59583333 -0.59166667 -0.5875 -0.58333333 -0.57916667 -0.575 -0.57083333 -0.56666667 -0.5625 -0.55833333 -0.55416667 -0.55 -0.54583333 -0.54166667 -0.5375 -0.53333333 -0.52916667 -0.525 -0.52083333 -0.51666667 -0.5125 -0.50833333 -0.50416667 -0.5 -0.49583333 -0.49166667 -0.4875 -0.48333333 -0.47916667 -0.475 -0.47083333 -0.46666667 -0.4625 -0.45833333 -0.45416667 -0.45 -0.44583333 -0.44166667 -0.4375 -0.43333333 -0.42916667 -0.425 -0.42083333 -0.41666667 -0.4125 -0.40833333 -0.40416667 -0.4 -0.39583333 -0.39166667 -0.3875 -0.38333333 -0.37916667 -0.375 -0.37083333 -0.36666667 -0.3625 -0.35833333 -0.35416667 -0.35 -0.34583333 -0.34166667 -0.3375 -0.33333333 -0.32916667 -0.325 -0.32083333 -0.31666667 -0.3125 -0.30833333 -0.30416667 -0.3 -0.29583333 -0.29166667 -0.2875 -0.28333333 -0.27916667 -0.275 -0.27083333 -0.26666667 -0.2625 -0.25833333 -0.25416667 -0.25 -0.24583333 -0.24166667 -0.2375 -0.23333333 -0.22916667 -0.225 -0.22083333 -0.21666667 -0.2125 -0.20833333 -0.20416667 -0.2 -0.19583333 -0.19166667 -0.1875 -0.18333333 -0.17916667 -0.175 -0.17083333 -0.16666667 -0.1625 -0.15833333 -0.15416667 -0.15 -0.14583333 -0.14166667 -0.1375 -0.13333333 -0.12916667 -0.125 -0.12083333 -0.11666667 -0.1125 -0.10833333 -0.10416667 -0.1 -0.09583333 -0.09166667 -0.0875 -0.08333333 -0.07916667 -0.075 -0.07083333 -0.06666667 -0.0625 -0.05833333 -0.05416667 -0.05 -0.04583333 -0.04166667 -0.0375 -0.03333333 -0.02916667 -0.025 -0.02083333 -0.01666667 -0.0125 -0.00833333 -0.00416667 0 0 0 0 0 0
  spline S101 degree 5 poles (30.7754, 3.7249) (30.7728, 3.7256) (30.7675, 3.7268) (30.7596, 3.7287) (30.7491, 3.7312) (30.736, 3.7343) (30.723, 3.7374) (30.7099, 3.7405) (30.6969, 3.7435) (30.6839, 3.7466) (30.671, 3.7496) (30.658, 3.7525) (30.6451, 3.7555) (30.6323, 3.7584) (30.6194, 3.7613) (30.6066, 3.7642) (30.5938, 3.767) (30.581, 3.7699) (30.5683, 3.7727) (30.5556, 3.7755) (30.5429, 3.7782) (30.5302, 3.781) (30.5176, 3.7837) (30.505, 3.7864) (30.4924, 3.7891) (30.4799, 3.7917) (30.4674, 3.7943) (30.4549, 3.797) (30.4424, 3.7995) (30.43, 3.8021) (30.4176, 3.8046) (30.4053, 3.8071) (30.3929, 3.8096) (30.3806, 3.8121) (30.3683, 3.8145) (30.3561, 3.817) (30.3439, 3.8194) (30.3317, 3.8217) (30.3195, 3.8241) (30.3074, 3.8264) (30.2953, 3.8288) (30.2832, 3.831) (30.2712, 3.8333) (30.2592, 3.8356) (30.2472, 3.8378) (30.2353, 3.84) (30.2233, 3.8422) (30.2115, 3.8443) (30.1996, 3.8464) (30.1878, 3.8486) (30.176, 3.8507) (30.1643, 3.8527) (30.1525, 3.8548) (30.1409, 3.8568) (30.1292, 3.8588) (30.1176, 3.8608) (30.106, 3.8628) (30.0944, 3.8647) (30.0829, 3.8666) (30.0714, 3.8685) (30.06, 3.8704) (30.0486, 3.8722) (30.0372, 3.8741) (30.0258, 3.8759) (30.0145, 3.8777) (30.0032, 3.8795) (29.992, 3.8812) (29.9807, 3.8829) (29.9696, 3.8846) (29.9584, 3.8863) (29.9473, 3.888) (29.9362, 3.8896) (29.9252, 3.8913) (29.9142, 3.8929) (29.9032, 3.8945) (29.8923, 3.896) (29.8814, 3.8976) (29.8705, 3.8991) (29.8597, 3.9006) (29.8489, 3.9021) (29.8382, 3.9035) (29.8274, 3.905) (29.8168, 3.9064) (29.8061, 3.9078) (29.7955, 3.9092) (29.785, 3.9106) (29.7744, 3.9119) (29.764, 3.9132) (29.7535, 3.9145) (29.7431, 3.9158) (29.7327, 3.9171) (29.7224, 3.9183) (29.7121, 3.9196) (29.7018, 3.9208) (29.6916, 3.922) (29.6814, 3.9231) (29.6713, 3.9243) (29.6612, 3.9254) (29.6512, 3.9265) (29.6411, 3.9276) (29.6312, 3.9287) (29.6212, 3.9297) (29.6113, 3.9308) (29.6015, 3.9318) (29.5917, 3.9328) (29.5819, 3.9338) (29.5722, 3.9348) (29.5625, 3.9357) (29.5529, 3.9366) (29.5433, 3.9375) (29.5337, 3.9384) (29.5242, 3.9393) (29.5147, 3.9402) (29.5053, 3.941) (29.4959, 3.9418) (29.4866, 3.9426) (29.4773, 3.9434) (29.468, 3.9442) (29.4588, 3.9449) (29.4497, 3.9457) (29.4406, 3.9464) (29.4315, 3.9471) (29.4225, 3.9478) (29.4135, 3.9484) (29.4045, 3.9491) (29.3957, 3.9497) (29.3868, 3.9503) (29.378, 3.9509) (29.3693, 3.9515) (29.3606, 3.9521) (29.3519, 3.9526) (29.3433, 3.9532) (29.3348, 3.9537) (29.3263, 3.9542) (29.3178, 3.9547) (29.3094, 3.9552) (29.301, 3.9556) (29.2927, 3.9561) (29.2845, 3.9565) (29.2763, 3.9569) (29.2681, 3.9573) (29.26, 3.9577) (29.2519, 3.9581) (29.2439, 3.9584) (29.236, 3.9588) (29.2281, 3.9591) (29.2202, 3.9594) (29.2124, 3.9597) (29.2047, 3.96) (29.197, 3.9603) (29.1893, 3.9605) (29.1817, 3.9607) (29.1742, 3.961) (29.1667, 3.9612) (29.1593, 3.9614) (29.1519, 3.9616) (29.1446, 3.9618) (29.1374, 3.9619) (29.1302, 3.9621) (29.123, 3.9622) (29.1159, 3.9623) (29.1089, 3.9625) (29.1019, 3.9626) (29.095, 3.9626) (29.0882, 3.9627) (29.0814, 3.9628) (29.0746, 3.9628) (29.068, 3.9629) (29.0613, 3.9629) (29.0548, 3.9629) (29.0483, 3.963) (29.0418, 3.963) (29.0355, 3.9629) (29.0291, 3.9629) (29.0229, 3.9629) (29.0167, 3.9629) (29.0106, 3.9628) (29.0045, 3.9627) (28.9985, 3.9627) (28.9926, 3.9626) (28.9867, 3.9625) (28.9809, 3.9624) (28.9752, 3.9623) (28.9695, 3.9622) (28.9639, 3.9621) (28.9584, 3.962) (28.9529, 3.9618) (28.9475, 3.9617) (28.9422, 3.9615) (28.9369, 3.9614) (28.9317, 3.9612) (28.9266, 3.961) (28.9215, 3.9609) (28.9166, 3.9607) (28.9117, 3.9605) (28.9068, 3.9603) (28.9021, 3.9601) (28.8974, 3.9599) (28.8928, 3.9597) (28.8882, 3.9595) (28.8838, 3.9593) (28.8794, 3.959) (28.8751, 3.9588) (28.8709, 3.9586) (28.8667, 3.9584) (28.8626, 3.9581) (28.8586, 3.9579) (28.8547, 3.9577) (28.8509, 3.9574) (28.8472, 3.9572) (28.8435, 3.9569) (28.8399, 3.9567) (28.8364, 3.9564) (28.833, 3.9562) (28.8297, 3.9559) (28.8264, 3.9557) (28.8233, 3.9555) (28.8202, 3.9552) (28.8172, 3.955) (28.8144, 3.9547) (28.8116, 3.9545) (28.8089, 3.9543) (28.8063, 3.954) (28.8037, 3.9538) (28.8013, 3.9536) (28.799, 3.9534) (28.7968, 3.9531) (28.7946, 3.9529) (28.7926, 3.9527) (28.7907, 3.9525) (28.7889, 3.9523) (28.7871, 3.9522) (28.7855, 3.952) (28.784, 3.9518) (28.7826, 3.9517) (28.7813, 3.9515) (28.7801, 3.9514) (28.779, 3.9512) (28.778, 3.9511) (28.7772, 3.951) (28.7764, 3.9509) (28.7759, 3.9509) (28.7756, 3.9508) (28.7754, 3.9508) (28.7753, 3.9508) knots -1 -1 -1 -1 -1 -1 -0.99583333 -0.99166667 -0.9875 -0.98333333 -0.97916667 -0.975 -0.97083333 -0.96666667 -0.9625 -0.95833333 -0.95416667 -0.95 -0.94583333 -0.94166667 -0.9375 -0.93333333 -0.92916667 -0.925 -0.92083333 -0.91666667 -0.9125 -0.90833333 -0.90416667 -0.9 -0.89583333 -0.89166667 -0.8875 -0.88333333 -0.87916667 -0.875 -0.87083333 -0.86666667 -0.8625 -0.85833333 -0.85416667 -0.85 -0.84583333 -0.84166667 -0.8375 -0.83333333 -0.82916667 -0.825 -0.82083333 -0.81666667 -0.8125 -0.80833333 -0.80416667 -0.8 -0.79583333 -0.79166667 -0.7875 -0.78333333 -0.77916667 -0.775 -0.77083333 -0.76666667 -0.7625 -0.75833333 -0.75416667 -0.75 -0.74583333 -0.74166667 -0.7375 -0.73333333 -0.72916667 -0.725 -0.72083333 -0.71666667 -0.7125 -0.70833333 -0.70416667 -0.7 -0.69583333 -0.69166667 -0.6875 -0.68333333 -0.67916667 -0.675 -0.67083333 -0.66666667 -0.6625 -0.65833333 -0.65416667 -0.65 -0.64583333 -0.64166667 -0.6375 -0.63333333 -0.62916667 -0.625 -0.62083333 -0.61666667 -0.6125 -0.60833333 -0.60416667 -0.6 -0.59583333 -0.59166667 -0.5875 -0.58333333 -0.57916667 -0.575 -0.57083333 -0.56666667 -0.5625 -0.55833333 -0.55416667 -0.55 -0.54583333 -0.54166667 -0.5375 -0.53333333 -0.52916667 -0.525 -0.52083333 -0.51666667 -0.5125 -0.50833333 -0.50416667 -0.5 -0.49583333 -0.49166667 -0.4875 -0.48333333 -0.47916667 -0.475 -0.47083333 -0.46666667 -0.4625 -0.45833333 -0.45416667 -0.45 -0.44583333 -0.44166667 -0.4375 -0.43333333 -0.42916667 -0.425 -0.42083333 -0.41666667 -0.4125 -0.40833333 -0.40416667 -0.4 -0.39583333 -0.39166667 -0.3875 -0.38333333 -0.37916667 -0.375 -0.37083333 -0.36666667 -0.3625 -0.35833333 -0.35416667 -0.35 -0.34583333 -0.34166667 -0.3375 -0.33333333 -0.32916667 -0.325 -0.32083333 -0.31666667 -0.3125 -0.30833333 -0.30416667 -0.3 -0.29583333 -0.29166667 -0.2875 -0.28333333 -0.27916667 -0.275 -0.27083333 -0.26666667 -0.2625 -0.25833333 -0.25416667 -0.25 -0.24583333 -0.24166667 -0.2375 -0.23333333 -0.22916667 -0.225 -0.22083333 -0.21666667 -0.2125 -0.20833333 -0.20416667 -0.2 -0.19583333 -0.19166667 -0.1875 -0.18333333 -0.17916667 -0.175 -0.17083333 -0.16666667 -0.1625 -0.15833333 -0.15416667 -0.15 -0.14583333 -0.14166667 -0.1375 -0.13333333 -0.12916667 -0.125 -0.12083333 -0.11666667 -0.1125 -0.10833333 -0.10416667 -0.1 -0.09583333 -0.09166667 -0.0875 -0.08333333 -0.07916667 -0.075 -0.07083333 -0.06666667 -0.0625 -0.05833333 -0.05416667 -0.05 -0.04583333 -0.04166667 -0.0375 -0.03333333 -0.02916667 -0.025 -0.02083333 -0.01666667 -0.0125 -0.00833333 -0.00416667 0 0 0 0 0 0
  line L197 (-18.7406, -22.1904) -> (-18.7401, -22.1898)
  line L198 (28.6734, 2.0967) -> (28.9671, 2.1182)
  spline S102 degree 5 poles (3.7249, -30.7754) (3.7256, -30.7728) (3.7268, -30.7675) (3.7287, -30.7596) (3.7312, -30.7491) (3.7343, -30.736) (3.7374, -30.723) (3.7405, -30.7099) (3.7435, -30.6969) (3.7466, -30.6839) (3.7496, -30.671) (3.7525, -30.658) (3.7555, -30.6451) (3.7584, -30.6323) (3.7613, -30.6194) (3.7642, -30.6066) (3.767, -30.5938) (3.7699, -30.581) (3.7727, -30.5683) (3.7755, -30.5556) (3.7782, -30.5429) (3.781, -30.5302) (3.7837, -30.5176) (3.7864, -30.505) (3.7891, -30.4924) (3.7917, -30.4799) (3.7943, -30.4674) (3.797, -30.4549) (3.7995, -30.4424) (3.8021, -30.43) (3.8046, -30.4176) (3.8071, -30.4053) (3.8096, -30.3929) (3.8121, -30.3806) (3.8145, -30.3683) (3.817, -30.3561) (3.8194, -30.3439) (3.8217, -30.3317) (3.8241, -30.3195) (3.8264, -30.3074) (3.8288, -30.2953) (3.831, -30.2832) (3.8333, -30.2712) (3.8356, -30.2592) (3.8378, -30.2472) (3.84, -30.2353) (3.8422, -30.2233) (3.8443, -30.2115) (3.8464, -30.1996) (3.8486, -30.1878) (3.8507, -30.176) (3.8527, -30.1643) (3.8548, -30.1525) (3.8568, -30.1409) (3.8588, -30.1292) (3.8608, -30.1176) (3.8628, -30.106) (3.8647, -30.0944) (3.8666, -30.0829) (3.8685, -30.0714) (3.8704, -30.06) (3.8722, -30.0486) (3.8741, -30.0372) (3.8759, -30.0258) (3.8777, -30.0145) (3.8795, -30.0032) (3.8812, -29.992) (3.8829, -29.9807) (3.8846, -29.9696) (3.8863, -29.9584) (3.888, -29.9473) (3.8896, -29.9362) (3.8913, -29.9252) (3.8929, -29.9142) (3.8945, -29.9032) (3.896, -29.8923) (3.8976, -29.8814) (3.8991, -29.8705) (3.9006, -29.8597) (3.9021, -29.8489) (3.9035, -29.8382) (3.905, -29.8274) (3.9064, -29.8168) (3.9078, -29.8061) (3.9092, -29.7955) (3.9106, -29.785) (3.9119, -29.7744) (3.9132, -29.764) (3.9145, -29.7535) (3.9158, -29.7431) (3.9171, -29.7327) (3.9183, -29.7224) (3.9196, -29.7121) (3.9208, -29.7018) (3.922, -29.6916) (3.9231, -29.6814) (3.9243, -29.6713) (3.9254, -29.6612) (3.9265, -29.6512) (3.9276, -29.6411) (3.9287, -29.6312) (3.9297, -29.6212) (3.9308, -29.6113) (3.9318, -29.6015) (3.9328, -29.5917) (3.9338, -29.5819) (3.9348, -29.5722) (3.9357, -29.5625) (3.9366, -29.5529) (3.9375, -29.5433) (3.9384, -29.5337) (3.9393, -29.5242) (3.9402, -29.5147) (3.941, -29.5053) (3.9418, -29.4959) (3.9426, -29.4866) (3.9434, -29.4773) (3.9442, -29.468) (3.9449, -29.4588) (3.9457, -29.4497) (3.9464, -29.4406) (3.9471, -29.4315) (3.9478, -29.4225) (3.9484, -29.4135) (3.9491, -29.4045) (3.9497, -29.3957) (3.9503, -29.3868) (3.9509, -29.378) (3.9515, -29.3693) (3.9521, -29.3606) (3.9526, -29.3519) (3.9532, -29.3433) (3.9537, -29.3348) (3.9542, -29.3263) (3.9547, -29.3178) (3.9552, -29.3094) (3.9556, -29.301) (3.9561, -29.2927) (3.9565, -29.2845) (3.9569, -29.2763) (3.9573, -29.2681) (3.9577, -29.26) (3.9581, -29.2519) (3.9584, -29.2439) (3.9588, -29.236) (3.9591, -29.2281) (3.9594, -29.2202) (3.9597, -29.2124) (3.96, -29.2047) (3.9603, -29.197) (3.9605, -29.1893) (3.9607, -29.1817) (3.961, -29.1742) (3.9612, -29.1667) (3.9614, -29.1593) (3.9616, -29.1519) (3.9618, -29.1446) (3.9619, -29.1374) (3.9621, -29.1302) (3.9622, -29.123) (3.9623, -29.1159) (3.9625, -29.1089) (3.9626, -29.1019) (3.9626, -29.095) (3.9627, -29.0882) (3.9628, -29.0814) (3.9628, -29.0746) (3.9629, -29.068) (3.9629, -29.0613) (3.9629, -29.0548) (3.963, -29.0483) (3.963, -29.0418) (3.9629, -29.0355) (3.9629, -29.0291) (3.9629, -29.0229) (3.9629, -29.0167) (3.9628, -29.0106) (3.9627, -29.0045) (3.9627, -28.9985) (3.9626, -28.9926) (3.9625, -28.9867) (3.9624, -28.9809) (3.9623, -28.9752) (3.9622, -28.9695) (3.9621, -28.9639) (3.962, -28.9584) (3.9618, -28.9529) (3.9617, -28.9475) (3.9615, -28.9422) (3.9614, -28.9369) (3.9612, -28.9317) (3.961, -28.9266) (3.9609, -28.9215) (3.9607, -28.9166) (3.9605, -28.9117) (3.9603, -28.9068) (3.9601, -28.9021) (3.9599, -28.8974) (3.9597, -28.8928) (3.9595, -28.8882) (3.9593, -28.8838) (3.959, -28.8794) (3.9588, -28.8751) (3.9586, -28.8709) (3.9584, -28.8667) (3.9581, -28.8626) (3.9579, -28.8586) (3.9577, -28.8547) (3.9574, -28.8509) (3.9572, -28.8472) (3.9569, -28.8435) (3.9567, -28.8399) (3.9564, -28.8364) (3.9562, -28.833) (3.9559, -28.8297) (3.9557, -28.8264) (3.9555, -28.8233) (3.9552, -28.8202) (3.955, -28.8172) (3.9547, -28.8144) (3.9545, -28.8116) (3.9543, -28.8089) (3.954, -28.8063) (3.9538, -28.8037) (3.9536, -28.8013) (3.9534, -28.799) (3.9531, -28.7968) (3.9529, -28.7946) (3.9527, -28.7926) (3.9525, -28.7907) (3.9523, -28.7889) (3.9522, -28.7871) (3.952, -28.7855) (3.9518, -28.784) (3.9517, -28.7826) (3.9515, -28.7813) (3.9514, -28.7801) (3.9512, -28.779) (3.9511, -28.778) (3.951, -28.7772) (3.9509, -28.7764) (3.9509, -28.7759) (3.9508, -28.7756) (3.9508, -28.7754) (3.9508, -28.7753) knots -1 -1 -1 -1 -1 -1 -0.99583333 -0.99166667 -0.9875 -0.98333333 -0.97916667 -0.975 -0.97083333 -0.96666667 -0.9625 -0.95833333 -0.95416667 -0.95 -0.94583333 -0.94166667 -0.9375 -0.93333333 -0.92916667 -0.925 -0.92083333 -0.91666667 -0.9125 -0.90833333 -0.90416667 -0.9 -0.89583333 -0.89166667 -0.8875 -0.88333333 -0.87916667 -0.875 -0.87083333 -0.86666667 -0.8625 -0.85833333 -0.85416667 -0.85 -0.84583333 -0.84166667 -0.8375 -0.83333333 -0.82916667 -0.825 -0.82083333 -0.81666667 -0.8125 -0.80833333 -0.80416667 -0.8 -0.79583333 -0.79166667 -0.7875 -0.78333333 -0.77916667 -0.775 -0.77083333 -0.76666667 -0.7625 -0.75833333 -0.75416667 -0.75 -0.74583333 -0.74166667 -0.7375 -0.73333333 -0.72916667 -0.725 -0.72083333 -0.71666667 -0.7125 -0.70833333 -0.70416667 -0.7 -0.69583333 -0.69166667 -0.6875 -0.68333333 -0.67916667 -0.675 -0.67083333 -0.66666667 -0.6625 -0.65833333 -0.65416667 -0.65 -0.64583333 -0.64166667 -0.6375 -0.63333333 -0.62916667 -0.625 -0.62083333 -0.61666667 -0.6125 -0.60833333 -0.60416667 -0.6 -0.59583333 -0.59166667 -0.5875 -0.58333333 -0.57916667 -0.575 -0.57083333 -0.56666667 -0.5625 -0.55833333 -0.55416667 -0.55 -0.54583333 -0.54166667 -0.5375 -0.53333333 -0.52916667 -0.525 -0.52083333 -0.51666667 -0.5125 -0.50833333 -0.50416667 -0.5 -0.49583333 -0.49166667 -0.4875 -0.48333333 -0.47916667 -0.475 -0.47083333 -0.46666667 -0.4625 -0.45833333 -0.45416667 -0.45 -0.44583333 -0.44166667 -0.4375 -0.43333333 -0.42916667 -0.425 -0.42083333 -0.41666667 -0.4125 -0.40833333 -0.40416667 -0.4 -0.39583333 -0.39166667 -0.3875 -0.38333333 -0.37916667 -0.375 -0.37083333 -0.36666667 -0.3625 -0.35833333 -0.35416667 -0.35 -0.34583333 -0.34166667 -0.3375 -0.33333333 -0.32916667 -0.325 -0.32083333 -0.31666667 -0.3125 -0.30833333 -0.30416667 -0.3 -0.29583333 -0.29166667 -0.2875 -0.28333333 -0.27916667 -0.275 -0.27083333 -0.26666667 -0.2625 -0.25833333 -0.25416667 -0.25 -0.24583333 -0.24166667 -0.2375 -0.23333333 -0.22916667 -0.225 -0.22083333 -0.21666667 -0.2125 -0.20833333 -0.20416667 -0.2 -0.19583333 -0.19166667 -0.1875 -0.18333333 -0.17916667 -0.175 -0.17083333 -0.16666667 -0.1625 -0.15833333 -0.15416667 -0.15 -0.14583333 -0.14166667 -0.1375 -0.13333333 -0.12916667 -0.125 -0.12083333 -0.11666667 -0.1125 -0.10833333 -0.10416667 -0.1 -0.09583333 -0.09166667 -0.0875 -0.08333333 -0.07916667 -0.075 -0.07083333 -0.06666667 -0.0625 -0.05833333 -0.05416667 -0.05 -0.04583333 -0.04166667 -0.0375 -0.03333333 -0.02916667 -0.025 -0.02083333 -0.01666667 -0.0125 -0.00833333 -0.00416667 0 0 0 0 0 0
  arc A104 (-10.0421, -29.3284) -> (-9.1146, -29.6298) centre (0, 0) ccw
  line L199 (-17.6281, -22.7115) -> (-17.8086, -22.9441)